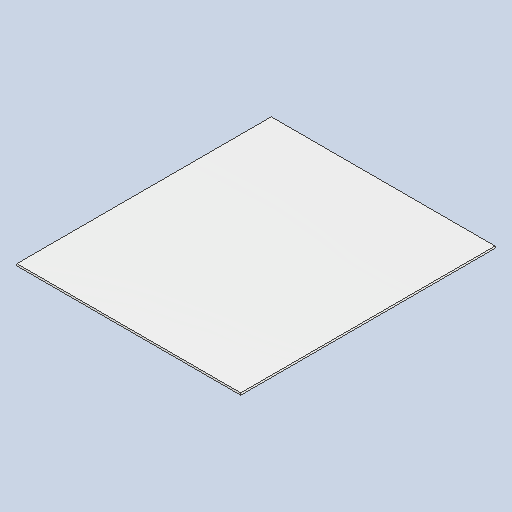
# Autodesk Inventor part: Base Acryl Plate
Saved by Autodesk Inventor 2023 (Build 270158000, 158)
## iProperties
Created: 2022-10-29
Part Number: Base Acryl Plate
Material: ABS Plastic
Document SubType Name: Modeling
Designer: chanh
Density: 1.06 g/cm^3
Appearance: Smooth - White
품번: 2
Author: chanh
Autodesk Inventor part; units mm, degrees
ref_plane "YZ Plane" through (0, 0, 0) normal (1, 0, 0) x (0, 1, 0)
ref_plane "XZ Plane" through (0, 0, 0) normal (0, 1, 0) x (-1, 0, 0)
ref_plane "XY Plane" through (0, 0, 0) normal (0, 0, 1) x (1, 0, 0)
sketch "Sketch1" plane through (0, 0, 0) normal (0, 1, 0) x (-1, 0, 0)
  line L0 (110, 125) -> (-110, 125)
  line L1 (-110, 125) -> (-110, -125)
  line L2 (-110, -125) -> (110, -125)
  line L3 (110, -125) -> (110, 125)
  line L4 (110, 125) -> (-110, -125) construction
  line L5 (-110, 125) -> (110, -125) construction
  point P0 (0, 0)
  dimension "d0" = 220
  dimension "d1" = 250
  constraints: 12 end point, 2 midpoint, 2 parallel, 1 horizontal, 1 perpendicular
  measures "d0" distance of L2.end L1.end
  measures "d1" distance of L1.end L0.end
extrude "Extrusion1" add sketch "Sketch1" along normal blind 2
body "Solid1"
